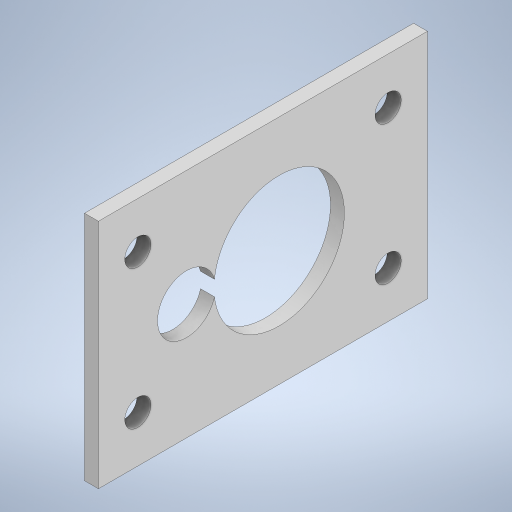
# Autodesk Inventor part: Base Top
Saved by Autodesk Inventor 2023 (Build 270158000, 158)
## iProperties
Created: 2023-02-13
Part Number: Base Top
Material: Generic
Document SubType Name: Modeling
Designer: tommy
Density: 1 g/cm^3
Appearance: Default
Author: tommy
Autodesk Inventor part; units mm, degrees
ref_plane "YZ Plane" through (0, 0, 0) normal (1, 0, 0) x (0, 1, 0)
ref_plane "XZ Plane" through (0, 0, 0) normal (0, 1, 0) x (-1, 0, 0)
ref_plane "XY Plane" through (0, 0, 0) normal (0, 0, 1) x (1, 0, 0)
sketch "Sketch1" plane through (0, 0, 0) normal (1, 0, 0) x (0, 1, 0)
  line L0 (0, 0) -> (12.7, 0)
  line L1 (12.7, 0) -> (12.7, -18.034)
  line L2 (12.7, -18.034) -> (0, -18.034)
  line L3 (0, -18.034) -> (0, 0)
  line L4 (-3.175, 0) -> (15.875, 0)
  line L5 (15.875, 0) -> (15.875, -18.034)
  line L6 (15.875, -18.034) -> (-3.175, -18.034)
  line L7 (-3.175, -18.034) -> (-3.175, 0)
  circle A0 centre (2.54, -15.875) radius 0.715
  circle A1 centre (2.548, -2.159) radius 0.715
  circle A2 centre (10.168, -2.159) radius 0.715
  circle A3 centre (10.16, -15.875) radius 0.715
  circle A4 centre (6.35, -9.906) radius 3.5719
  circle A5 centre (6.35, -4.826) radius 1.5875
  point P0 (6.35, 0)
  point P1 (6.765, -6.3583)
  point P2 (5.935, -6.3583)
  dimension "d0" = 12.7
  dimension "d1" = 18.034
  dimension "d2" = 19.05
  dimension "d3" = 3.175
  dimension "d5" = 1.43
  dimension "d9" = 13.716
  dimension "d10" = 7.62
  dimension "d11" = 7.62
  dimension "d12" = 13.716
  dimension "d13" = 2.54
  dimension "d20" = 7.1437
  dimension "d21" = 3.175
  dimension "d23" = 2.159
  dimension "d24" = 2.159
  constraints: 16 end point, 6 centre point, 4 parallel, 3 equal radius, 2 horizontal, 2 perpendicular, 1 midpoint
  measures "d0" distance of L1.end L2.end
  measures "d1" distance of L0.end L1.end
  measures "d2" distance of L5.end L6.end
  measures "d3" distance between parallel lines of L3 L7
  measures "d5" diameter of A0
  measures "d9" distance of A1.centre A0.centre
  measures "d10" distance of A3.centre A0.centre
  measures "d11" distance of A1.centre A2.centre
  measures "d12" distance of A3.centre A2.centre
  measures "d13" distance from line of L3 A0.centre
  measures "d20" diameter of A4
  measures "d21" diameter of A5
  measures "d23" distance from line of L2 A0.centre
  measures "d24" vertical distance of L1.end A3.centre
extrude "Extrusion1" add sketch "Sketch1" along normal blind 0.762 contours L0 L1 L2 L3
body "Solid1"
